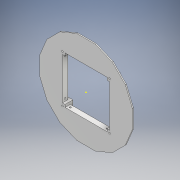
# Autodesk Inventor part: composite_base
Saved by Autodesk Inventor 2017 (Build 210142000, 142)
## iProperties
Created: 2018-12-08
Part Number: composite_base
Material: ABS Plastic
Document SubType Name: Modeling
Designer: simulator
Density: 1.06 g/cm^3
Appearance: Smooth - White
Mass: 53.348 g
Surface Area: 434.091 cm^2
Volume: 50.3283 cm^3
Author: simulator
## iProperties of the stored document composite_base_3DPrint.ipt
Created: 2019-03-18
Part Number: composite_base_3DPrint
Material: Generic
Document SubType Name: Modeling
Designer: simulator
Density: 1 g/cm^3
Appearance: Default
Author: simulator
Autodesk Inventor part; units mm, degrees
ref_plane "YZ Plane" through (0, 0, 0) normal (1, 0, 0) x (0, 1, 0)
sketch "Sketch1" plane through (0, 0, 0) normal (0, 0, 1) x (1, 0, 0)
  point P0 (0, 0)
sketch "Sketch2" plane through (0, 0, 0) normal (0, 1, 0) x (-1, 0, 0)
  line L0 (40, 40) -> (-40, 40)
  line L1 (-40, 40) -> (-40, -40)
  line L2 (-40, -40) -> (40, -40)
  line L3 (40, -40) -> (40, 40)
  line L4 (50, 50) -> (-50, 50)
  line L5 (-50, 50) -> (-50, -50)
  line L6 (-50, -50) -> (50, -50)
  line L7 (50, -50) -> (50, 50)
  line L8 (50, 50) -> (40, 50)
  line L9 (40, 50) -> (40, 40)
  line L10 (40, 40) -> (50, 40)
  line L11 (50, 40) -> (50, 50)
  line L12 (40, -40) -> (50, -40)
  line L13 (50, -40) -> (50, -50)
  line L14 (50, -50) -> (40, -50)
  line L15 (40, -50) -> (40, -40)
  line L16 (-50, -50) -> (-40, -50)
  line L17 (-40, -50) -> (-40, -40)
  line L18 (-40, -40) -> (-50, -40)
  line L19 (-50, -40) -> (-50, -50)
  line L20 (-50, 50) -> (-40, 50)
  line L21 (-40, 50) -> (-40, 40)
  line L22 (-40, 40) -> (-50, 40)
  line L23 (-50, 40) -> (-50, 50)
  line L24 (-50, 40) -> (-45, 40)
  line L25 (-45, 40) -> (-45, -40)
  line L26 (-45, -40) -> (-50, -40)
  line L27 (-50, -40) -> (-50, 40)
  line L28 (-40, 45) -> (40, 45)
  line L29 (40, 45) -> (40, 50)
  line L30 (40, 50) -> (-40, 50)
  line L31 (-40, 50) -> (-40, 45)
  line L32 (50, 40) -> (45, 40)
  line L33 (45, 40) -> (45, -40)
  line L34 (45, -40) -> (50, -40)
  line L35 (50, -40) -> (50, 40)
  line L36 (-40, -45) -> (40, -45)
  line L37 (40, -45) -> (40, -50)
  line L38 (40, -50) -> (-40, -50)
  line L39 (-40, -50) -> (-40, -45)
  line L40 (-50, 50) -> (-40, 50)
  line L41 (-40, 50) -> (-40, 40)
  line L42 (-40, 40) -> (-50, 40)
  line L43 (-50, 40) -> (-50, 50)
  line L44 (-40, -50) -> (40, -50)
  line L45 (40, -50) -> (40, -45)
  line L46 (40, -45) -> (-40, -45)
  line L47 (-40, -45) -> (-40, -50)
  line L48 (-40, -40) -> (40, 40)
  point P0 (-50, 0)
  point P1 (-50, 0)
  point P2 (0, 0)
  point P3 (0, 0)
  dimension "d0" = 80
  dimension "d1" = 80
  dimension "d2" = 10
  constraints: 98 end point, 24 parallel, 12 perpendicular, 11 horizontal, 6 midpoint, 2 coincident, 4 other
  measures "d0" distance of L2.end L0.start
  measures "d1" distance of L1.end L2.end
  measures "d2" distance between parallel lines of L3 L7
extrude "Extrusion1" add sketch "Sketch2" along normal blind 100 contours L9 L4 L7 L10 | L22 L5 L4 L21 | L12 L7 L6 L15 | L17 L6 L5 L18
extrude "Extrusion2" add sketch "Sketch2" along normal blind 10 contours L28 L21 L4 L9 | L10 L7 L12 L33 | L25 L18 L5 L22 | L15 L6 L17 L36
sketch "Sketch3" plane through (0, 100, 0) normal (0, 1, 0) x (1, 0, 0)
  line L0 (50, -40) -> (50, 40) projected
  line L1 (45, 40) -> (50, 40) projected
  line L2 (45, 40) -> (45, -40) projected
  line L3 (50, -40) -> (45, -40) projected
  line L4 (-40, -50) -> (40, -50) projected
  line L5 (40, -45) -> (40, -50) projected
  line L6 (40, -45) -> (-40, -45) projected
  line L7 (-40, -50) -> (-40, -45) projected
  line L8 (-50, 40) -> (-45, 40) projected
  line L9 (-50, 40) -> (-50, -40) projected
  line L10 (-45, -40) -> (-50, -40) projected
  line L11 (-45, -40) -> (-45, 40) projected
  line L12 (40, 50) -> (-40, 50) projected
  line L13 (-40, 45) -> (-40, 50) projected
  line L14 (-40, 45) -> (40, 45) projected
  line L15 (40, 50) -> (40, 45) projected
  point P0 (0, 0)
extrude "Extrusion3" add sketch "Sketch3" against normal blind 10
sketch "Sketch4" plane through (50, 100, -50) normal (0, 0, -1) x (-1, 0, 0)
  line L0 (90, -90) -> (90, -10) projected
  line L1 (10, -90) -> (90, -90) projected
  line L2 (10, -90) -> (10, -10) projected
  line L3 (90, -10) -> (10, -10) projected
  line L4 (0, 0) -> (100, 0) projected
  line L5 (0, -100) -> (0, 0) projected
  line L6 (0, -100) -> (100, -100) projected
  line L7 (100, -100) -> (100, 0) projected
  line L8 (90, -10) -> (10, -10) projected
  line L9 (10, -10) -> (15, -10)
  line L10 (15, -10) -> (20, -10)
  line L11 (15, -10) -> (15, -5)
  line L12 (90, -10) -> (85, -10)
  line L13 (85, -10) -> (85, -5)
  line L14 (10, -90) -> (15, -90)
  line L15 (90, -90) -> (10, -90) projected
  line L16 (15, -90) -> (20, -90)
  line L17 (15, -90) -> (15, -95)
  line L18 (90, -90) -> (90, -10) projected
  line L19 (90, -90) -> (85, -90)
  line L20 (85, -90) -> (85, -95)
  point P0 (50, -100)
  dimension "d9" = 5
  dimension "d10" = 5
  dimension "d11" = 5
  dimension "d12" = 5
  dimension "d13" = 5
  dimension "d14" = 5
  dimension "d15" = 5
  dimension "d16" = 5
  dimension "d17" = 5
  dimension "d18" = 5
  constraints: 20 end point, 6 point on line, 4 coincident, 3 perpendicular, 1 vertical
  measures "d9" distance of L2.end L9.end
  measures "d10" distance of L9.end L10.end
  measures "d11" distance of L9.end L11.end
  measures "d12" distance of L0.end L12.end
  measures "d13" distance of L12.end L13.end
  measures "d14" distance of L1.start L14.end
  measures "d15" distance of L14.end L16.end
  measures "d16" distance of L14.end L17.end
  measures "d17" distance of L0.start L19.end
  measures "d18" distance of L19.end L20.end
hole "Hole1" at (35, 95, -50) at (-35, 95, -50) at (-35, 5, -50) at (35, 5, -50) direction (0, 0, 1) diameter 3 depth 100 tip angle 118
sketch "Sketch5" plane through (-50, 0, -50) normal (-1, 0, 0) x (0, 0, 1)
  line L0 (90, 10) -> (90, 90)
  line L1 (10, 10) -> (90, 10)
  line L2 (10, 10) -> (10, 90)
  line L3 (90, 90) -> (10, 90)
  line L4 (0, 100) -> (100, 100)
  line L5 (0, 0) -> (0, 100)
  line L6 (0, 0) -> (100, 0)
  line L7 (100, 0) -> (100, 100)
  line L8 (90, 90) -> (10, 90)
  line L9 (10, 90) -> (15, 90)
  line L10 (15, 90) -> (20, 90)
  line L11 (15, 90) -> (15, 95)
  line L12 (90, 90) -> (85, 90)
  line L13 (85, 90) -> (85, 95)
  line L14 (10, 10) -> (15, 10)
  line L15 (90, 10) -> (10, 10)
  line L16 (15, 10) -> (20, 10)
  line L17 (15, 10) -> (15, 5)
  line L18 (90, 10) -> (90, 90)
  line L19 (90, 10) -> (85, 10)
  line L20 (85, 10) -> (85, 5)
  point P0 (50, 0)
  point P1 (0, 0)
  dimension "d26" = 5
  dimension "d27" = 5
  dimension "d28" = 5
  dimension "d29" = 5
  dimension "d30" = 5
  dimension "d31" = 5
  dimension "d32" = 5
  dimension "d33" = 5
  dimension "d34" = 5
  dimension "d35" = 5
  constraints: 42 end point, 6 point on line, 4 coincident, 3 perpendicular, 1 vertical
  measures "d26" distance of L2.end L9.end
  measures "d27" distance of L9.end L10.end
  measures "d28" distance of L9.end L11.end
  measures "d29" distance of L0.end L12.end
  measures "d30" distance of L12.end L13.end
  measures "d31" distance of L1.start L14.end
  measures "d32" distance of L14.end L16.end
  measures "d33" distance of L14.end L17.end
  measures "d34" distance of L0.start L19.end
  measures "d35" distance of L19.end L20.end
hole "Hole2" at (-50, 95, -35) at (-50, 95, 35) at (-50, 5, 35) at (-50, 5, -35) direction (1, 0, 0) diameter 3 depth 100 tip angle 118
sketch "Sketch9" plane through (0, 100, 0) normal (0, 1, 0) x (1, 0, 0)
  line L0 (50, 50) -> (-50, 50) projected
  line L1 (50, 50) -> (40, 40)
  line L2 (50, -50) -> (40, -40)
  line L3 (-50, -50) -> (-40, -40)
  line L4 (-50, 50) -> (-40, 40)
  point P0 (0, 0)
  point P1 (-45, 45)
  point P2 (45, 45)
  point P3 (45, -45)
  point P4 (-45, -45)
  constraints: 8 end point, 4 midpoint
hole "Hole3" at (45, 100, -45) at (-45, 100, -45) at (-45, 100, 45) at (45, 100, 45) direction (0, -1, 0) diameter 3 depth 8 tip angle 118
sketch "Sketch10" plane through (0, 0, 0) normal (0, -1, 0) x (1, 0, 0)
  line L0 (50, 50) -> (-50, 50)
  line L1 (50, 50) -> (40, 40)
  line L2 (50, -50) -> (40, -40)
  line L3 (-50, -50) -> (-40, -40)
  line L4 (-50, 50) -> (-40, 40)
  point P0 (0, 0)
  point P1 (0, 0)
  point P2 (-45, 45)
  point P3 (45, 45)
  point P4 (45, -45)
  point P5 (-45, -45)
  constraints: 10 end point, 4 midpoint
hole "Hole4" at (-45, 0, -45) at (45, 0, -45) at (45, 0, 45) at (-45, 0, 45) direction (0, 1, 0) diameter 3 depth 8 tip angle 118
sketch "Sketch11" plane through (40, 0, -40) normal (0, 0, 1) x (1, 0, 0)
  point P0 (-40, 0)
sketch "Sketch13" plane through (0, 100, 0) normal (0, 1, 0) x (1, 0, 0)
  line L0 (-22.6221, 49.1489) -> (20.7989, 49.1489) construction
  line L1 (20.7989, 49.1489) -> (20.7989, 45.013) construction
  line L2 (20.7989, 45.013) -> (-22.6221, 45.013) construction
  line L3 (-22.6221, 45.013) -> (-22.6221, 49.1489) construction
  line L4 (-18.345, 49.0751) -> (-19.2242, 45.5751)
  line L5 (-19.2242, 45.5751) -> (-19.7461, 45.5751)
  line L6 (-19.7461, 45.5751) -> (-20.458, 48.4795)
  line L7 (-20.458, 48.4795) -> (-21.1501, 45.5751)
  line L8 (-21.1501, 45.5751) -> (-21.6663, 45.5751)
  line L9 (-21.6663, 45.5751) -> (-22.5597, 49.0751)
  line L10 (-22.5597, 49.0751) -> (-22.0804, 49.0751)
  line L11 (-22.0804, 49.0751) -> (-21.377, 46.1736)
  line L12 (-21.377, 46.1736) -> (-20.6793, 49.0751)
  line L13 (-20.6793, 49.0751) -> (-20.2056, 49.0751)
  line L14 (-20.2056, 49.0751) -> (-19.5022, 46.1395)
  line L15 (-19.5022, 46.1395) -> (-18.8016, 49.0751)
  line L16 (-18.8016, 49.0751) -> (-18.345, 49.0751)
  line L17 (-16.7084, 45.5751) -> (-18.0642, 45.5751)
  line L18 (-18.0642, 45.5751) -> (-18.0642, 45.9325)
  line L19 (-18.0642, 45.9325) -> (-17.6189, 45.9325)
  line L20 (-17.6189, 45.9325) -> (-17.6189, 48.7177)
  line L21 (-17.6189, 48.7177) -> (-18.0642, 48.7177)
  line L22 (-18.0642, 48.7177) -> (-18.0642, 49.0751)
  line L23 (-18.0642, 49.0751) -> (-16.7084, 49.0751)
  line L24 (-16.7084, 49.0751) -> (-16.7084, 48.7177)
  line L25 (-16.7084, 48.7177) -> (-17.1537, 48.7177)
  line L26 (-17.1537, 48.7177) -> (-17.1537, 45.9325)
  line L27 (-17.1537, 45.9325) -> (-16.7084, 45.9325)
  line L28 (-16.7084, 45.9325) -> (-16.7084, 45.5751)
  line L29 (-14.1047, 45.5751) -> (-16.1327, 45.5751)
  line L30 (-16.1327, 45.5751) -> (-16.1327, 49.0751)
  line L31 (-16.1327, 49.0751) -> (-15.6675, 49.0751)
  line L32 (-15.6675, 49.0751) -> (-15.6675, 45.9892)
  line L33 (-15.6675, 45.9892) -> (-14.1047, 45.9892)
  line L34 (-14.1047, 45.9892) -> (-14.1047, 45.5751)
  line L35 (-11.2883, 49.0751) -> (-12.471, 47.1237)
  line L36 (-12.471, 47.1237) -> (-12.471, 45.5751)
  line L37 (-12.471, 45.5751) -> (-12.9362, 45.5751)
  line L38 (-12.9362, 45.5751) -> (-12.9362, 47.0755)
  line L39 (-12.9362, 47.0755) -> (-14.1189, 49.0751)
  line L40 (-14.1189, 49.0751) -> (-13.6027, 49.0751)
  line L41 (-13.6027, 49.0751) -> (-12.7007, 47.535)
  line L42 (-12.7007, 47.535) -> (-11.7818, 49.0751)
  line L43 (-11.7818, 49.0751) -> (-11.2883, 49.0751)
  line L44 (-11.3421, 45.5751) -> (-10.1622, 49.0751)
  line L45 (-10.1622, 49.0751) -> (-9.5893, 49.0751)
  line L46 (-9.5893, 49.0751) -> (-8.4094, 45.5751)
  line L47 (-8.4094, 45.5751) -> (-8.9001, 45.5751)
  line L48 (-8.9001, 45.5751) -> (-9.2178, 46.5536)
  line L49 (-9.2178, 46.5536) -> (-10.5537, 46.5536)
  line L50 (-10.5537, 46.5536) -> (-10.8713, 45.5751)
  line L51 (-10.8713, 45.5751) -> (-11.3421, 45.5751)
  line L52 (-9.3454, 46.9507) -> (-9.8871, 48.5986)
  line L53 (-9.8871, 48.5986) -> (-10.426, 46.9507)
  line L54 (-10.426, 46.9507) -> (-9.3454, 46.9507)
  line L55 (-5.3689, 45.5751) -> (-5.973, 45.5751)
  line L56 (-5.973, 45.5751) -> (-7.0792, 46.9677)
  line L57 (-7.0792, 46.9677) -> (-7.6124, 46.9677)
  line L58 (-7.6124, 46.9677) -> (-7.6124, 45.5751)
  line L59 (-7.6124, 45.5751) -> (-8.0776, 45.5751)
  line L60 (-8.0776, 45.5751) -> (-8.0776, 49.0751)
  line L61 (-8.0776, 49.0751) -> (-7.1756, 49.0751)
  spline S0 degree 2 poles (-7.1756, 49.0751) (-6.875, 49.0751) (-6.4694, 49.0099) (-6.285, 48.8908) knots 0 0 0 1 2 2 2
  spline S1 degree 2 poles (-6.285, 48.8908) (-6.1007, 48.7716) (-5.8879, 48.4001) (-5.8879, 48.125) knots 0 0 0 1 2 2 2
  spline S2 degree 2 poles (-5.8879, 48.125) (-5.8879, 47.7421) (-6.2793, 47.223) (-6.614, 47.0982) knots 0 0 0 1 2 2 2
  line L62 (-6.614, 47.0982) -> (-5.3689, 45.5751)
  spline S3 degree 2 poles (-6.3729, 48.0881) (-6.3729, 48.2412) (-6.4807, 48.4767) (-6.5942, 48.5532) knots 0 0 0 1 2 2 2
  spline S4 degree 2 poles (-6.5942, 48.5532) (-6.6934, 48.6185) (-6.9572, 48.6724) (-7.1501, 48.6724) knots 0 0 0 1 2 2 2
  line L63 (-7.1501, 48.6724) -> (-7.6124, 48.6724)
  line L64 (-7.6124, 48.6724) -> (-7.6124, 47.3563)
  line L65 (-7.6124, 47.3563) -> (-7.204, 47.3563)
  spline S5 degree 2 poles (-7.204, 47.3563) (-7.0026, 47.3563) (-6.6821, 47.4272) (-6.5715, 47.5378) knots 0 0 0 1 2 2 2
  spline S6 degree 2 poles (-6.5715, 47.5378) (-6.4694, 47.6343) (-6.3729, 47.9066) (-6.3729, 48.0881) knots 0 0 0 1 2 2 2
  line L66 (-4.2741, 45.5751) -> (-4.2741, 48.661)
  line L67 (-4.2741, 48.661) -> (-5.4483, 48.661)
  line L68 (-5.4483, 48.661) -> (-5.4483, 49.0751)
  line L69 (-5.4483, 49.0751) -> (-2.6347, 49.0751)
  line L70 (-2.6347, 49.0751) -> (-2.6347, 48.661)
  line L71 (-2.6347, 48.661) -> (-3.8089, 48.661)
  line L72 (-3.8089, 48.661) -> (-3.8089, 45.5751)
  line L73 (-3.8089, 45.5751) -> (-4.2741, 45.5751)
  line L74 (-1.0605, 45.5751) -> (-2.4163, 45.5751)
  line L75 (-2.4163, 45.5751) -> (-2.4163, 45.9325)
  line L76 (-2.4163, 45.9325) -> (-1.971, 45.9325)
  line L77 (-1.971, 45.9325) -> (-1.971, 48.7177)
  line L78 (-1.971, 48.7177) -> (-2.4163, 48.7177)
  line L79 (-2.4163, 48.7177) -> (-2.4163, 49.0751)
  line L80 (-2.4163, 49.0751) -> (-1.0605, 49.0751)
  line L81 (-1.0605, 49.0751) -> (-1.0605, 48.7177)
  line L82 (-1.0605, 48.7177) -> (-1.5058, 48.7177)
  line L83 (-1.5058, 48.7177) -> (-1.5058, 45.9325)
  line L84 (-1.5058, 45.9325) -> (-1.0605, 45.9325)
  line L85 (-1.0605, 45.9325) -> (-1.0605, 45.5751)
  line L86 (3.5598, 45.5751) -> (3.0946, 45.5751)
  line L87 (3.0946, 45.5751) -> (3.0946, 47.2882)
  line L88 (3.0946, 47.2882) -> (1.4836, 47.2882)
  line L89 (1.4836, 47.2882) -> (1.4836, 45.5751)
  line L90 (1.4836, 45.5751) -> (1.0185, 45.5751)
  line L91 (1.0185, 45.5751) -> (1.0185, 49.0751)
  line L92 (1.0185, 49.0751) -> (1.4836, 49.0751)
  line L93 (1.4836, 49.0751) -> (1.4836, 47.7023)
  line L94 (1.4836, 47.7023) -> (3.0946, 47.7023)
  line L95 (3.0946, 47.7023) -> (3.0946, 49.0751)
  line L96 (3.0946, 49.0751) -> (3.5598, 49.0751)
  line L97 (3.5598, 49.0751) -> (3.5598, 45.5751)
  spline S7 degree 2 poles (6.745, 48.6752) (6.9435, 48.4426) (7.1647, 47.7619) (7.1647, 47.3251) knots 0 0 0 1 2 2 2
  spline S8 degree 2 poles (7.1647, 47.3251) (7.1647, 46.8997) (6.9492, 46.2105) (6.745, 45.9779) knots 0 0 0 1 2 2 2
  spline S9 degree 2 poles (6.745, 45.9779) (6.5294, 45.734) (5.9593, 45.5014) (5.6161, 45.5014) knots 0 0 0 1 2 2 2
  spline S10 degree 2 poles (5.6161, 45.5014) (5.2616, 45.5014) (4.6943, 45.7425) (4.4873, 45.9779) knots 0 0 0 1 2 2 2
  spline S11 degree 2 poles (4.4873, 45.9779) (4.2859, 46.2105) (4.0703, 46.894) (4.0703, 47.3251) knots 0 0 0 1 2 2 2
  spline S12 degree 2 poles (4.0703, 47.3251) (4.0703, 47.7647) (4.2887, 48.4341) (4.4901, 48.6752) knots 0 0 0 1 2 2 2
  spline S13 degree 2 poles (4.4901, 48.6752) (4.6943, 48.9078) (5.2644, 49.1489) (5.6161, 49.1489) knots 0 0 0 1 2 2 2
  spline S14 degree 2 poles (5.6161, 49.1489) (5.9735, 49.1489) (6.5464, 48.8993) (6.745, 48.6752) knots 0 0 0 1 2 2 2
  spline S15 degree 2 poles (6.6797, 47.3251) (6.6797, 47.6712) (6.5294, 48.2072) (6.3933, 48.3831) knots 0 0 0 1 2 2 2
  spline S16 degree 2 poles (6.3933, 48.3831) (6.2543, 48.5646) (5.8629, 48.7461) (5.619, 48.7461) knots 0 0 0 1 2 2 2
  spline S17 degree 2 poles (5.619, 48.7461) (5.3665, 48.7461) (4.9865, 48.5703) (4.8418, 48.3831) knots 0 0 0 1 2 2 2
  spline S18 degree 2 poles (4.8418, 48.3831) (4.7028, 48.2044) (4.5553, 47.6655) (4.5553, 47.3251) knots 0 0 0 1 2 2 2
  spline S19 degree 2 poles (4.5553, 47.3251) (4.5553, 46.6359) (5.1339, 45.9041) (5.619, 45.9041) knots 0 0 0 1 2 2 2
  spline S20 degree 2 poles (5.619, 45.9041) (6.104, 45.9041) (6.6797, 46.6359) (6.6797, 47.3251) knots 0 0 0 1 2 2 2
  line L98 (11.5979, 49.0751) -> (10.7186, 45.5751)
  line L99 (10.7186, 45.5751) -> (10.1968, 45.5751)
  line L100 (10.1968, 45.5751) -> (9.4848, 48.4795)
  line L101 (9.4848, 48.4795) -> (8.7928, 45.5751)
  line L102 (8.7928, 45.5751) -> (8.2766, 45.5751)
  line L103 (8.2766, 45.5751) -> (7.3831, 49.0751)
  line L104 (7.3831, 49.0751) -> (7.8625, 49.0751)
  line L105 (7.8625, 49.0751) -> (8.5659, 46.1736)
  line L106 (8.5659, 46.1736) -> (9.2636, 49.0751)
  line L107 (9.2636, 49.0751) -> (9.7373, 49.0751)
  line L108 (9.7373, 49.0751) -> (10.4407, 46.1395)
  line L109 (10.4407, 46.1395) -> (11.1412, 49.0751)
  line L110 (11.1412, 49.0751) -> (11.5979, 49.0751)
  line L111 (11.6376, 45.5751) -> (12.8175, 49.0751)
  line L112 (12.8175, 49.0751) -> (13.3904, 49.0751)
  line L113 (13.3904, 49.0751) -> (14.5703, 45.5751)
  line L114 (14.5703, 45.5751) -> (14.0797, 45.5751)
  line L115 (14.0797, 45.5751) -> (13.762, 46.5536)
  line L116 (13.762, 46.5536) -> (12.4261, 46.5536)
  line L117 (12.4261, 46.5536) -> (12.1084, 45.5751)
  line L118 (12.1084, 45.5751) -> (11.6376, 45.5751)
  line L119 (13.6344, 46.9507) -> (13.0926, 48.5986)
  line L120 (13.0926, 48.5986) -> (12.5537, 46.9507)
  line L121 (12.5537, 46.9507) -> (13.6344, 46.9507)
  line L122 (17.6109, 45.5751) -> (17.0067, 45.5751)
  line L123 (17.0067, 45.5751) -> (15.9006, 46.9677)
  line L124 (15.9006, 46.9677) -> (15.3673, 46.9677)
  line L125 (15.3673, 46.9677) -> (15.3673, 45.5751)
  line L126 (15.3673, 45.5751) -> (14.9022, 45.5751)
  line L127 (14.9022, 45.5751) -> (14.9022, 49.0751)
  line L128 (14.9022, 49.0751) -> (15.8041, 49.0751)
  spline S21 degree 2 poles (15.8041, 49.0751) (16.1048, 49.0751) (16.5104, 49.0099) (16.6947, 48.8908) knots 0 0 0 1 2 2 2
  spline S22 degree 2 poles (16.6947, 48.8908) (16.8791, 48.7716) (17.0918, 48.4001) (17.0918, 48.125) knots 0 0 0 1 2 2 2
  spline S23 degree 2 poles (17.0918, 48.125) (17.0918, 47.7421) (16.7004, 47.223) (16.3657, 47.0982) knots 0 0 0 1 2 2 2
  line L129 (16.3657, 47.0982) -> (17.6109, 45.5751)
  spline S24 degree 2 poles (16.6068, 48.0881) (16.6068, 48.2412) (16.499, 48.4767) (16.3856, 48.5532) knots 0 0 0 1 2 2 2
  spline S25 degree 2 poles (16.3856, 48.5532) (16.2863, 48.6185) (16.0225, 48.6724) (15.8297, 48.6724) knots 0 0 0 1 2 2 2
  line L130 (15.8297, 48.6724) -> (15.3673, 48.6724)
  line L131 (15.3673, 48.6724) -> (15.3673, 47.3563)
  line L132 (15.3673, 47.3563) -> (15.7758, 47.3563)
  spline S26 degree 2 poles (15.7758, 47.3563) (15.9771, 47.3563) (16.2976, 47.4272) (16.4083, 47.5378) knots 0 0 0 1 2 2 2
  spline S27 degree 2 poles (16.4083, 47.5378) (16.5104, 47.6343) (16.6068, 47.9066) (16.6068, 48.0881) knots 0 0 0 1 2 2 2
  spline S28 degree 2 poles (20.6485, 47.3223) (20.6485, 46.8429) (20.26, 46.0715) (19.9338, 45.8559) knots 0 0 0 1 2 2 2
  spline S29 degree 2 poles (19.9338, 45.8559) (19.6672, 45.6886) (19.1198, 45.5751) (18.6943, 45.5751) knots 0 0 0 1 2 2 2
  line L133 (18.6943, 45.5751) -> (17.8888, 45.5751)
  line L134 (17.8888, 45.5751) -> (17.8888, 49.0751)
  line L135 (17.8888, 49.0751) -> (18.6858, 49.0751)
  spline S30 degree 2 poles (18.6858, 49.0751) (19.1793, 49.0751) (19.7409, 48.9276) (19.9395, 48.7972) knots 0 0 0 1 2 2 2
  spline S31 degree 2 poles (19.9395, 48.7972) (20.277, 48.5731) (20.6485, 47.8328) (20.6485, 47.3223) knots 0 0 0 1 2 2 2
  spline S32 degree 2 poles (20.1635, 47.328) (20.1635, 47.7307) (19.8969, 48.3008) (19.6331, 48.4625) knots 0 0 0 1 2 2 2
  spline S33 degree 2 poles (19.6331, 48.4625) (19.4459, 48.5731) (19.0233, 48.6724) (18.7085, 48.6724) knots 0 0 0 1 2 2 2
  line L136 (18.7085, 48.6724) -> (18.354, 48.6724)
  line L137 (18.354, 48.6724) -> (18.354, 45.9779)
  line L138 (18.354, 45.9779) -> (18.7085, 45.9779)
  spline S34 degree 2 poles (18.7085, 45.9779) (19.0177, 45.9779) (19.4856, 46.0771) (19.6757, 46.2105) knots 0 0 0 1 2 2 2
  spline S35 degree 2 poles (19.6757, 46.2105) (19.9196, 46.375) (20.1635, 46.9195) (20.1635, 47.328) knots 0 0 0 1 2 2 2
  point P0 (0, 0)
  constraints: 2 other
extrude "Extrusion7" cut sketch "Sketch13" against normal blind 0.4
ref_plane "Work Plane1" through (0, 20, 0) normal (0, 1, 0) x (1, 0, 0)
sketch "Sketch14" plane through (0, 20, 0) normal (0, 1, 0) x (1, 0, 0)
  line L0 (-40, -45) -> (-40, -50) projected
  line L1 (36.5, -50) -> (36.5, -45) projected
  line L2 (40, -50) -> (40, -45) projected
  line L3 (40, -45) -> (-40, -45) projected
  line L4 (-50, -50) -> (50, -50) projected
  line L5 (-45, -40) -> (-45, 40) projected
  line L6 (-50, -40) -> (-45, -40) projected
  line L7 (-50, 50) -> (-50, -50) projected
  line L8 (-45, 40) -> (-50, 40) projected
  line L9 (-40, 50) -> (-40, 45) projected
  line L10 (50, 50) -> (-50, 50) projected
  line L11 (-40, 45) -> (40, 45) projected
  line L12 (40, 45) -> (40, 50) projected
  line L13 (50, -50) -> (50, 50) projected
  line L14 (50, 40) -> (45, 40) projected
  line L15 (45, 40) -> (45, -40) projected
  line L16 (45, -40) -> (50, -40) projected
  point P0 (0, 0)
extrude "Extrusion8" add sketch "Sketch14" along normal blind 0.4 contours L3 L1 L4 L0 | L3 L2 L4 L1 | L7 L8 L5 L6 | L16 L15 L14 L13 | L10 L12 L11 L9
pattern_linear "Rectangular Pattern1" count 7 spacing 10 along (0, 1, 0) of "Extrusion8"
sketch "Sketch15" plane through (0, 100, 0) normal (0, 1, 0) x (1, 0, 0)
  line L0 (18.6943, 45.5751) -> (17.8888, 45.5751) projected
  line L1 (17.8888, 45.5751) -> (17.8888, 49.0751) projected
  line L2 (17.8888, 49.0751) -> (18.6858, 49.0751) projected
  line L3 (16.3657, 47.0982) -> (17.6109, 45.5751) projected
  line L4 (17.6109, 45.5751) -> (17.0067, 45.5751) projected
  line L5 (17.0067, 45.5751) -> (15.9006, 46.9677) projected
  line L6 (15.9006, 46.9677) -> (15.3673, 46.9677) projected
  line L7 (15.3673, 46.9677) -> (15.3673, 45.5751) projected
  line L8 (15.3673, 45.5751) -> (14.9022, 45.5751) projected
  line L9 (14.9022, 45.5751) -> (14.9022, 49.0751) projected
  line L10 (14.9022, 49.0751) -> (15.8041, 49.0751) projected
  line L11 (12.1084, 45.5751) -> (11.6376, 45.5751) projected
  line L12 (11.6376, 45.5751) -> (12.8175, 49.0751) projected
  line L13 (12.8175, 49.0751) -> (13.3904, 49.0751) projected
  line L14 (13.3904, 49.0751) -> (14.5703, 45.5751) projected
  line L15 (14.5703, 45.5751) -> (14.0797, 45.5751) projected
  line L16 (14.0797, 45.5751) -> (13.762, 46.5536) projected
  line L17 (13.762, 46.5536) -> (12.4261, 46.5536) projected
  line L18 (12.4261, 46.5536) -> (12.1084, 45.5751) projected
  line L19 (3.5598, 49.0751) -> (3.5598, 45.5751) projected
  line L20 (3.5598, 45.5751) -> (3.0946, 45.5751) projected
  line L21 (3.0946, 45.5751) -> (3.0946, 47.2882) projected
  line L22 (3.0946, 47.2882) -> (1.4836, 47.2882) projected
  line L23 (1.4836, 47.2882) -> (1.4836, 45.5751) projected
  line L24 (1.4836, 45.5751) -> (1.0185, 45.5751) projected
  line L25 (1.0185, 45.5751) -> (1.0185, 49.0751) projected
  line L26 (1.0185, 49.0751) -> (1.4836, 49.0751) projected
  line L27 (1.4836, 49.0751) -> (1.4836, 47.7023) projected
  line L28 (1.4836, 47.7023) -> (3.0946, 47.7023) projected
  line L29 (3.0946, 47.7023) -> (3.0946, 49.0751) projected
  line L30 (3.0946, 49.0751) -> (3.5598, 49.0751) projected
  line L31 (-3.8089, 45.5751) -> (-4.2741, 45.5751) projected
  line L32 (-4.2741, 45.5751) -> (-4.2741, 48.661) projected
  line L33 (-4.2741, 48.661) -> (-5.4483, 48.661) projected
  line L34 (-5.4483, 48.661) -> (-5.4483, 49.0751) projected
  line L35 (-5.4483, 49.0751) -> (-2.6347, 49.0751) projected
  line L36 (-2.6347, 49.0751) -> (-2.6347, 48.661) projected
  line L37 (-2.6347, 48.661) -> (-3.8089, 48.661) projected
  line L38 (-3.8089, 48.661) -> (-3.8089, 45.5751) projected
  line L39 (-6.614, 47.0982) -> (-5.3689, 45.5751) projected
  line L40 (-5.3689, 45.5751) -> (-5.973, 45.5751) projected
  line L41 (-5.973, 45.5751) -> (-7.0792, 46.9677) projected
  line L42 (-7.0792, 46.9677) -> (-7.6124, 46.9677) projected
  line L43 (-7.6124, 46.9677) -> (-7.6124, 45.5751) projected
  line L44 (-7.6124, 45.5751) -> (-8.0776, 45.5751) projected
  line L45 (-8.0776, 45.5751) -> (-8.0776, 49.0751) projected
  line L46 (-8.0776, 49.0751) -> (-7.1756, 49.0751) projected
  line L47 (-10.8713, 45.5751) -> (-11.3421, 45.5751) projected
  line L48 (-11.3421, 45.5751) -> (-10.1622, 49.0751) projected
  line L49 (-10.1622, 49.0751) -> (-9.5893, 49.0751) projected
  line L50 (-9.5893, 49.0751) -> (-8.4094, 45.5751) projected
  line L51 (-8.4094, 45.5751) -> (-8.9001, 45.5751) projected
  line L52 (-8.9001, 45.5751) -> (-9.2178, 46.5536) projected
  line L53 (-9.2178, 46.5536) -> (-10.5537, 46.5536) projected
  line L54 (-10.5537, 46.5536) -> (-10.8713, 45.5751) projected
  line L55 (-14.1047, 45.9892) -> (-14.1047, 45.5751) projected
  line L56 (-14.1047, 45.5751) -> (-16.1327, 45.5751) projected
  line L57 (-16.1327, 45.5751) -> (-16.1327, 49.0751) projected
  line L58 (-16.1327, 49.0751) -> (-15.6675, 49.0751) projected
  line L59 (-15.6675, 49.0751) -> (-15.6675, 45.9892) projected
  line L60 (-15.6675, 45.9892) -> (-14.1047, 45.9892) projected
  line L61 (-18.8016, 49.0751) -> (-18.345, 49.0751) projected
  line L62 (-18.345, 49.0751) -> (-19.2242, 45.5751) projected
  line L63 (-19.2242, 45.5751) -> (-19.7461, 45.5751) projected
  line L64 (-19.7461, 45.5751) -> (-20.458, 48.4795) projected
  line L65 (-20.458, 48.4795) -> (-21.1501, 45.5751) projected
  line L66 (-21.1501, 45.5751) -> (-21.6663, 45.5751) projected
  line L67 (-21.6663, 45.5751) -> (-22.5597, 49.0751) projected
  line L68 (-22.5597, 49.0751) -> (-22.0804, 49.0751) projected
  line L69 (-22.0804, 49.0751) -> (-21.377, 46.1736) projected
  line L70 (-21.377, 46.1736) -> (-20.6793, 49.0751) projected
  line L71 (-20.6793, 49.0751) -> (-20.2056, 49.0751) projected
  line L72 (-20.2056, 49.0751) -> (-19.5022, 46.1395) projected
  line L73 (-19.5022, 46.1395) -> (-18.8016, 49.0751) projected
  line L74 (-16.7084, 45.9325) -> (-16.7084, 45.5751) projected
  line L75 (-16.7084, 45.5751) -> (-18.0642, 45.5751) projected
  line L76 (-18.0642, 45.5751) -> (-18.0642, 45.9325) projected
  line L77 (-18.0642, 45.9325) -> (-17.6189, 45.9325) projected
  line L78 (-17.6189, 45.9325) -> (-17.6189, 48.7177) projected
  line L79 (-17.6189, 48.7177) -> (-18.0642, 48.7177) projected
  line L80 (-18.0642, 48.7177) -> (-18.0642, 49.0751) projected
  line L81 (-18.0642, 49.0751) -> (-16.7084, 49.0751) projected
  line L82 (-16.7084, 49.0751) -> (-16.7084, 48.7177) projected
  line L83 (-16.7084, 48.7177) -> (-17.1537, 48.7177) projected
  line L84 (-17.1537, 48.7177) -> (-17.1537, 45.9325) projected
  line L85 (-17.1537, 45.9325) -> (-16.7084, 45.9325) projected
  line L86 (-11.7818, 49.0751) -> (-11.2883, 49.0751) projected
  line L87 (-11.2883, 49.0751) -> (-12.471, 47.1237) projected
  line L88 (-12.471, 47.1237) -> (-12.471, 45.5751) projected
  line L89 (-12.471, 45.5751) -> (-12.9362, 45.5751) projected
  line L90 (-12.9362, 45.5751) -> (-12.9362, 47.0755) projected
  line L91 (-12.9362, 47.0755) -> (-14.1189, 49.0751) projected
  line L92 (-14.1189, 49.0751) -> (-13.6027, 49.0751) projected
  line L93 (-13.6027, 49.0751) -> (-12.7007, 47.535) projected
  line L94 (-12.7007, 47.535) -> (-11.7818, 49.0751) projected
  line L95 (-1.0605, 45.9325) -> (-1.0605, 45.5751) projected
  line L96 (-1.0605, 45.5751) -> (-2.4163, 45.5751) projected
  line L97 (-2.4163, 45.5751) -> (-2.4163, 45.9325) projected
  line L98 (-2.4163, 45.9325) -> (-1.971, 45.9325) projected
  line L99 (-1.971, 45.9325) -> (-1.971, 48.7177) projected
  line L100 (-1.971, 48.7177) -> (-2.4163, 48.7177) projected
  line L101 (-2.4163, 48.7177) -> (-2.4163, 49.0751) projected
  line L102 (-2.4163, 49.0751) -> (-1.0605, 49.0751) projected
  line L103 (-1.0605, 49.0751) -> (-1.0605, 48.7177) projected
  line L104 (-1.0605, 48.7177) -> (-1.5058, 48.7177) projected
  line L105 (-1.5058, 48.7177) -> (-1.5058, 45.9325) projected
  line L106 (-1.5058, 45.9325) -> (-1.0605, 45.9325) projected
  line L107 (11.1412, 49.0751) -> (11.5979, 49.0751) projected
  line L108 (11.5979, 49.0751) -> (10.7186, 45.5751) projected
  line L109 (10.7186, 45.5751) -> (10.1968, 45.5751) projected
  line L110 (10.1968, 45.5751) -> (9.4848, 48.4795) projected
  line L111 (9.4848, 48.4795) -> (8.7928, 45.5751) projected
  line L112 (8.7928, 45.5751) -> (8.2766, 45.5751) projected
  line L113 (8.2766, 45.5751) -> (7.3831, 49.0751) projected
  line L114 (7.3831, 49.0751) -> (7.8625, 49.0751) projected
  line L115 (7.8625, 49.0751) -> (8.5659, 46.1736) projected
  line L116 (8.5659, 46.1736) -> (9.2636, 49.0751) projected
  line L117 (9.2636, 49.0751) -> (9.7373, 49.0751) projected
  line L118 (9.7373, 49.0751) -> (10.4407, 46.1395) projected
  line L119 (10.4407, 46.1395) -> (11.1412, 49.0751) projected
  circle A0 centre (-45, -45) radius 1.5 projected
  circle A1 centre (45, 45) radius 1.5 projected
  circle A2 centre (-45, 45) radius 1.5 projected
  circle A3 centre (45, -45) radius 1.5 projected
  line L120 (-50, 50) -> (-50, -50) projected
  line L121 (-50, -50) -> (50, -50) projected
  line L122 (50, -50) -> (50, 50) projected
  line L123 (50, 50) -> (-50, 50) projected
  line L124 (-45, -40) -> (-45, 40) projected
  line L125 (-45, 40) -> (-40, 40) projected
  line L126 (-40, 40) -> (-40, 45) projected
  line L127 (-40, 45) -> (40, 45) projected
  line L128 (40, 45) -> (40, 40) projected
  line L129 (40, 40) -> (45, 40) projected
  line L130 (45, 40) -> (45, -40) projected
  line L131 (45, -40) -> (40, -40) projected
  line L132 (40, -40) -> (40, -45) projected
  line L133 (40, -45) -> (-40, -45) projected
  line L134 (-40, -45) -> (-40, -40) projected
  line L135 (-40, -40) -> (-45, -40) projected
  point P0 (0, 0)
  point P1 (19.9395, 48.7972)
  point P2 (20.6485, 47.3223)
  point P3 (19.9338, 45.8559)
  point P4 (16.6947, 48.8908)
  point P5 (17.0918, 48.125)
  point P6 (-6.285, 48.8908)
  point P7 (-5.8879, 48.125)
  point P8 (5.6161, 49.1489)
  point P9 (6.745, 48.6752)
  point P10 (7.1647, 47.3251)
  point P11 (6.745, 45.9779)
  point P12 (5.6161, 45.5014)
  point P13 (4.4873, 45.9779)
  point P14 (4.0703, 47.3251)
  point P15 (4.4901, 48.6752)
  constraints: 18 other
ref_plane "Work Plane2" through (-30, 0, -40) normal (1, 0, 0) x (0, 0, -1)
sketch "Sketch17" plane through (-30, 0, -40) normal (1, 0, 0) x (0, 0, -1)
  line L0 (5, 80.4) -> (10, 80.4) projected
  line L1 (10, 80.4) -> (10, 90) projected
  line L2 (10, 90) -> (5, 90) projected
  line L3 (5, 90) -> (5, 100) projected
  line L4 (0, 100) -> (5, 100) projected
  line L5 (0, 0) -> (0, 100) projected
  line L6 (0, 0) -> (5, 0) projected
  line L7 (5, 0) -> (5, 10) projected
  line L8 (5, 10) -> (10, 10) projected
  line L9 (10, 10) -> (10, 20) projected
  line L10 (10, 20) -> (5, 20) projected
  line L11 (5, 20) -> (5, 20.4) projected
  line L12 (5, 20.4) -> (10, 20.4) projected
  line L13 (10, 20.4) -> (10, 30) projected
  line L14 (10, 30) -> (5, 30) projected
  line L15 (5, 30) -> (5, 30.4) projected
  line L16 (5, 30.4) -> (10, 30.4) projected
  line L17 (10, 30.4) -> (10, 40) projected
  line L18 (10, 40) -> (5, 40) projected
  line L19 (5, 40) -> (5, 40.4) projected
  line L20 (5, 40.4) -> (10, 40.4) projected
  line L21 (10, 40.4) -> (10, 50) projected
  line L22 (10, 50) -> (5, 50) projected
  line L23 (5, 50) -> (5, 50.4) projected
  line L24 (5, 50.4) -> (10, 50.4) projected
  line L25 (10, 50.4) -> (10, 60) projected
  line L26 (10, 60) -> (5, 60) projected
  line L27 (5, 60) -> (5, 60.4) projected
  line L28 (5, 60.4) -> (10, 60.4) projected
  line L29 (10, 60.4) -> (10, 70) projected
  line L30 (10, 70) -> (5, 70) projected
  line L31 (5, 70) -> (5, 70.4) projected
  line L32 (5, 70.4) -> (10, 70.4) projected
  line L33 (10, 70.4) -> (10, 80) projected
  line L34 (10, 80) -> (5, 80) projected
  line L35 (5, 80) -> (5, 80.4) projected
  line L36 (0, 90) -> (10, 90)
  line L37 (10, 90) -> (10, 10)
  line L38 (5, 10) -> (10, 10) projected
  line L39 (10, 90) -> (5, 90)
  line L40 (5, 90) -> (5, 10)
  line L41 (5, 10) -> (10, 10)
  line L42 (10, 10) -> (10, 90)
  point P0 (-40, 0)
  constraints: 12 end point, 2 parallel, 1 horizontal, 1 perpendicular, 1 point on line
sketch "Sketch18" plane through (-30, 0, -40) normal (1, 0, 0) x (0, 0, -1)
  line L0 (5, 10) -> (10, 10) projected
  line L1 (10, 90) -> (5, 90) projected
  line L2 (10, 90) -> (5, 90)
  line L3 (5, 90) -> (5, 10)
  line L4 (5, 10) -> (10, 10)
  line L5 (10, 10) -> (10, 90)
  point P0 (-40, 0)
  constraints: 8 end point, 2 parallel, 1 horizontal, 1 perpendicular
extrude "Extrusion10" add sketch "Sketch18" along normal blind 0.4
pattern_linear "Rectangular Pattern2" count 7 spacing 10 along (1, 0, 0) of "Extrusion10"
pattern_circular "Circular Pattern2" count 4 over 360 about axis through (0, -10, 0) along (0, 1, 0) of "Extrusion10", "Rectangular Pattern2"
sketch "Sketch19" plane through (0, 100, 0) normal (0, 1, 0) x (1, 0, 0)
  line L0 (-102.8827, 70.81) -> (90.8034, 70.81)
  line L1 (90.8034, 70.81) -> (90.8034, -74.3505)
  line L2 (90.8034, -74.3505) -> (-102.8827, -74.3505)
  line L3 (-102.8827, -74.3505) -> (-102.8827, 70.81)
  point P0 (0, 0)
  constraints: 8 end point, 2 parallel, 1 horizontal, 1 perpendicular
extrude "Extrusion11" cut sketch "Sketch19" against normal up to surface (90 mm away)
sketch "Sketch20" plane through (0, 10, 0) normal (0, 1, 0) x (1, 0, 0)
  line L0 (-50, -50) -> (50, -50) projected
  line L1 (50, 50) -> (50, -50) projected
  line L2 (-50, 50) -> (50, 50) projected
  line L3 (-50, -50) -> (-50, 50) projected
  line L4 (40, -45) -> (-40, -45) projected
  line L5 (-40, -40) -> (-40, -45) projected
  line L6 (-45, -40) -> (-40, -40) projected
  line L7 (-45, -40) -> (-45, 40) projected
  line L8 (-40, 40) -> (-45, 40) projected
  line L9 (-40, 45) -> (-40, 40) projected
  line L10 (-40, 45) -> (40, 45) projected
  line L11 (40, 40) -> (40, 45) projected
  line L12 (45, 40) -> (40, 40) projected
  line L13 (45, 40) -> (45, -40) projected
  line L14 (40, -40) -> (45, -40) projected
  line L15 (40, -45) -> (40, -40) projected
  line L16 (-40, 40) -> (-50, 50)
  line L17 (50, -50) -> (50, 50) projected
  line L18 (45, 40) -> (40, 40) projected
  line L19 (50, 50) -> (40, 40)
  line L20 (-40, -40) -> (-45, -40) projected
  line L21 (-50, -50) -> (-40, -40)
  line L22 (50, -50) -> (40, -40)
  circle A0 centre (-45, -45) radius 1.5 projected
  circle A1 centre (45, 45) radius 1.5 projected
  point P0 (0, 0)
  point P1 (-45, 45)
  point P2 (45, -45)
  constraints: 8 end point, 2 coincident, 2 midpoint, 1 perpendicular
hole "Hole5" at (-45, 10, -45) at (-45, 10, 45) at (45, 10, 45) at (45, 10, -45) direction (0, -1, 0) diameter 3 depth 20 tip angle 118
sketch "Sketch21" plane through (40, 0, 45) normal (0, 0, -1) x (-1, 0, 0)
  point P0 (40, 0)
sketch "Sketch22" plane through (0, 0, 0) normal (0, -1, 0) x (1, 0, 0)
  line L0 (-36.5, 50) -> (-36.5, 45) projected
  circle A0 centre (45, 45) radius 1.5 projected
  circle A1 centre (-45, -45) radius 1.5 projected
  circle A2 centre (45, -45) radius 1.5 projected
  circle A3 centre (-45, 45) radius 1.5 projected
  line L1 (-50, 50) -> (50, 50) projected
  line L2 (-50, -50) -> (-50, 50) projected
  line L3 (50, -50) -> (-50, -50) projected
  line L4 (50, 50) -> (50, -50) projected
  line L5 (40, 45) -> (-40, 45) projected
  line L6 (40, 40) -> (40, 45) projected
  line L7 (45, 40) -> (40, 40) projected
  line L8 (45, -40) -> (45, 40) projected
  line L9 (40, -40) -> (45, -40) projected
  line L10 (40, -45) -> (40, -40) projected
  line L11 (-40, -45) -> (40, -45) projected
  line L12 (-40, -40) -> (-40, -45) projected
  line L13 (-45, -40) -> (-40, -40) projected
  line L14 (-45, 40) -> (-45, -40) projected
  line L15 (-40, 40) -> (-45, 40) projected
  line L16 (-40, 45) -> (-40, 40) projected
  point P0 (0, 0)
sketch "Sketch23" plane through (-50, 0, 50) normal (0, 0, 1) x (1, 0, 0)
  circle A0 centre (15, 5) radius 1.5 projected
  circle A1 centre (85, 5) radius 1.5 projected
  line L0 (0, 10) -> (100, 10) projected
  line L1 (0, 0) -> (0, 10) projected
  line L2 (0, 0) -> (100, 0) projected
  line L3 (100, 0) -> (100, 10) projected
  point P0 (50, 0)
sketch "Sketch24" plane through (0, 0, 0) normal (0, -1, 0) x (1, 0, 0)
  circle A0 centre (0, 0) radius 90
  line L0 (-50, 50) -> (50, 50) projected
  line L1 (-50, -50) -> (-50, 50) projected
  line L2 (50, 50) -> (50, -50) projected
  line L3 (50, -50) -> (-50, -50) projected
  dimension "d104" = 180
  constraints: 1 centre point, 1 coincident
  measures "d104" diameter of A0
extrude "Extrusion12" add sketch "Sketch24" against normal blind 2
sketch "Sketch25" plane through (0, 0, 0) normal (0, -1, 0) x (1, 0, 0)
  line L0 (-88.2707, -17.5581) -> (-88.2707, 17.5581)
  line L1 (-88.2707, 17.5581) -> (-74.8323, 50.0013)
  line L2 (-74.8323, 50.0013) -> (-50.0013, 74.8323)
  line L3 (-50.0013, 74.8323) -> (-17.5581, 88.2707)
  line L4 (-17.5581, 88.2707) -> (17.5581, 88.2707)
  line L5 (17.5581, 88.2707) -> (50.0013, 74.8323)
  line L6 (50.0013, 74.8323) -> (74.8323, 50.0013)
  line L7 (74.8323, 50.0013) -> (88.2707, 17.5581)
  line L8 (88.2707, 17.5581) -> (88.2707, -17.5581)
  line L9 (88.2707, -17.5581) -> (74.8323, -50.0013)
  line L10 (74.8323, -50.0013) -> (50.0013, -74.8323)
  line L11 (50.0013, -74.8323) -> (17.5581, -88.2707)
  line L12 (17.5581, -88.2707) -> (-17.5581, -88.2707)
  line L13 (-17.5581, -88.2707) -> (-50.0013, -74.8323)
  line L14 (-50.0013, -74.8323) -> (-74.8323, -50.0013)
  line L15 (-74.8323, -50.0013) -> (-88.2707, -17.5581)
  line L16 (0, 0) -> (-31.7308, 0)
  circle A0 centre (0, 0) radius 115.722
  dimension "d109" = 180
  constraints: 34 end point, 2 coincident, 1 centre point, 1 horizontal, 1 parallel, 33 other
  measures "d109" distance of L0.start L7.end
extrude "Extrusion13" cut sketch "Sketch25" against normal blind 10
sketch "Sketch27" plane through (0, 10, 0) normal (0, 1, 0) x (1, 0, 0)
  circle A0 centre (45, -45) radius 1.5 projected
  circle A1 centre (-45, 45) radius 1.5 projected
  circle A2 centre (-45, -45) radius 1.5 projected
  circle A3 centre (45, 45) radius 1.5 projected
  line L0 (-50, -50) -> (50, -50) projected
  line L1 (50, 50) -> (50, -50) projected
  line L2 (-50, 50) -> (50, 50) projected
  line L3 (-50, -50) -> (-50, 50) projected
  line L4 (40, -45) -> (-40, -45) projected
  line L5 (-40, -40) -> (-40, -45) projected
  line L6 (-45, -40) -> (-40, -40) projected
  line L7 (-45, -40) -> (-45, 40) projected
  line L8 (-40, 40) -> (-45, 40) projected
  line L9 (-40, 45) -> (-40, 40) projected
  line L10 (-40, 45) -> (40, 45) projected
  line L11 (40, 40) -> (40, 45) projected
  line L12 (45, 40) -> (40, 40) projected
  line L13 (45, 40) -> (45, -40) projected
  line L14 (40, -40) -> (45, -40) projected
  line L15 (40, -45) -> (40, -40) projected
  line L16 (-40, -40) -> (-45, -40) projected
  line L17 (-50, -50) -> (-40, -50)
  line L18 (-40, -50) -> (-40, -40)
  line L19 (-40, -40) -> (-50, -40)
  line L20 (-50, -40) -> (-50, -50)
  line L21 (-50, 50) -> (-50, -50) projected
  line L22 (-50, 50) -> (-40, 50)
  line L23 (-40, 50) -> (-40, 40)
  line L24 (-40, 40) -> (-50, 40)
  line L25 (-50, 40) -> (-50, 50)
  line L26 (50, 50) -> (40, 50)
  line L27 (40, 50) -> (40, 40)
  line L28 (40, 40) -> (50, 40)
  line L29 (50, 40) -> (50, 50)
  line L30 (50, 50) -> (50, -50) projected
  line L31 (40, -45) -> (40, -40) projected
  line L32 (50, -50) -> (40, -50)
  line L33 (40, -50) -> (40, -40)
  line L34 (40, -40) -> (50, -40)
  line L35 (50, -40) -> (50, -50)
  point P0 (0, 0)
  constraints: 32 end point, 8 parallel, 4 horizontal, 4 perpendicular
extrude "Extrusion15" add sketch "Sketch27" along normal blind 5 contours L3 L19 L6 L5 L18 L0 | L33 L15 L14 L34 L1 L0 | L3 L2 L23 L9 L8 L24 | L28 L12 L11 L27 L2 L1
body "Solid1"
